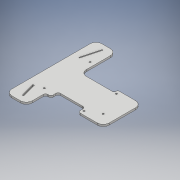
# Autodesk Inventor part: battery_mount
Saved by Autodesk Inventor 2017.2 (Build 212233000, 233)
## iProperties
Created: 2017-09-20
Part Number: battery_mount
Material: Generic
Document SubType Name: Modeling
Designer: Nic
Density: 1 g/cm^3
Appearance: Default
Author: Nic
Autodesk Inventor part; units mm, degrees
ref_plane "YZ Plane" through (0, 0, 0) normal (1, 0, 0) x (0, 1, 0)
ref_plane "XZ Plane" through (0, 0, 0) normal (0, 1, 0) x (-1, 0, 0)
ref_plane "XY Plane" through (0, 0, 0) normal (0, 0, 1) x (1, 0, 0)
sketch "Sketch1" plane through (0, 0, 0) normal (0, 0, 1) x (1, 0, 0)
  line L0 (-34, 30) -> (-34, -100)
  line L1 (96, -68) -> (96, -24)
  line L2 (0, -10) -> (0, 30)
  line L3 (-10, 40) -> (-24, 40)
  circle A0 centre (78, -60) radius 1.3
  circle A1 centre (-7.65, 3.7) radius 1.3
  arc A2 (-24, 40) -> (-34, 30) centre (-24, 30) ccw
  arc A3 (0, 30) -> (-10, 40) centre (-10, 30) ccw
  arc A4 (86, -78) -> (96, -68) centre (86, -68) ccw
  line L4 (0, -82) -> (0, -100)
  line L5 (-10, -110) -> (-24, -110)
  arc A5 (-10, -110) -> (0, -100) centre (-10, -100) ccw
  arc A6 (-34, -100) -> (-24, -110) centre (-24, -100) ccw
  line L6 (59, -14) -> (86, -14)
  arc A7 (96, -24) -> (86, -14) centre (86, -24) ccw
  line L7 (54, -74) -> (54, -70)
  line L8 (50, -66) -> (13, -66)
  line L9 (9, -70) -> (9, -72)
  line L10 (5, -78) -> (4, -78)
  line L11 (58, -78) -> (86, -78)
  arc A8 (13, -66) -> (9, -70) centre (13, -70) ccw
  arc A9 (54, -74) -> (58, -78) centre (58, -74) ccw
  arc A10 (54, -70) -> (50, -66) centre (50, -70) ccw
  line L12 (-16.3182, -100.6212) -> (-22.7887, -76.473)
  line L13 (-22.7887, -76.473) -> (-20.4705, -75.8519)
  line L14 (-20.4705, -75.8519) -> (-14, -100)
  line L15 (-14, -100) -> (-16.3182, -100.6212)
  line L16 (-10, -100) -> (-24, -100) construction
  line L17 (-34, -35) -> (96, -35) construction
  line L18 (-15.5455, 32) -> (-23.8277, 1.0904)
  line L19 (-15.5455, 32) -> (-14, 31.5859)
  line L20 (-14, 31.5859) -> (-22.2822, 0.6763)
  line L21 (-22.2822, 0.6763) -> (-23.8277, 1.0904)
  line L22 (53, -20) -> (10, -20)
  line L23 (56, -17) -> (56, -17)
  arc A11 (53, -20) -> (56, -17) centre (53, -17) ccw
  arc A12 (59, -14) -> (56, -17) centre (59, -17) ccw
  arc A13 (0, -10) -> (10, -20) centre (10, -10) ccw
  line L24 (-10, 30) -> (-24, 30) construction
  circle A14 centre (60, -20) radius 1.3
  circle A15 centre (58, -72) radius 1.3
  line L25 (9, -72) -> (9, -74)
  arc A16 (5, -78) -> (9, -74) centre (5, -74) ccw
  arc A17 (4, -78) -> (0, -82) centre (4, -82) ccw
  circle A18 centre (-8, -72) radius 1.3
  line L26 (58, -72) -> (-8, -72) construction
  point P0 (0, 0)
  point P1 (-34, 40)
  point P2 (0, 40)
  point P3 (-34, -110)
  point P4 (96, -14)
  point P5 (9, -78)
  point P6 (0, -20)
  point P7 (54, -66)
  point P8 (9, -66)
  dimension "d2" = 2.6
  dimension "d4" = 18
  dimension "d5" = 40
  dimension "d7" = 34
  dimension "d10" = 26.35
  dimension "d14" = 10
  dimension "d23" = 10
  dimension "d25" = 17.7
  dimension "d27" = 45
  dimension "d29" = 64
  dimension "d31" = 32
  dimension "d32" = 12
  dimension "d33" = 130
  dimension "d36" = 4
  dimension "d38" = 2.4
  dimension "d39" = 75
  dimension "d42" = 42
  dimension "d46" = 1.6
  dimension "d48" = 6
  dimension "d49" = 3
  dimension "d50" = 10
  dimension "d51" = 75
  dimension "d52" = 32
  dimension "d55" = 8
  dimension "d56" = 14
  dimension "d57" = 25
  dimension "d58" = 14
  dimension "d59" = 40
  dimension "d60" = 18
  dimension "d61" = 20
  dimension "d62" = 12
  dimension "d63" = 20
  dimension "d64" = 100
  dimension "d65" = 4
  dimension "d66" = 60
  dimension "d67" = 4
  dimension "d68" = 66
  constraints: 54 end point, 29 tangent, 28 point on circle, 19 centre point, 19 point on line, 16 perpendicular, 11 equal radius, 4 vertical, 3 horizontal, 1 collinear, 1 midpoint
  measures "d2" diameter of A0
  measures "d4" distance from line of L1 A0.centre
  measures "d5" distance from line of L3 point (0, 0)
  measures "d7" distance of point (0, 40) point (-34, 40)
  measures "d10" distance from line of L0 A1.centre
  measures "d14" radius of A2
  measures "d23" radius of A7
  measures "d25" distance from line of L6 A1.centre
  measures "d27" distance of point (54, -66) point (9, -66)
  measures "d29" distance between parallel lines of L6 L10
  measures "d31" distance from line of L5.start L10
  measures "d32" distance between parallel lines of L11 L8
  measures "d33" distance between parallel lines of L0 L1
  measures "d36" radius of A9
  measures "d38" distance between parallel lines of L14 L12
  measures "d39" angle of L12 L16
  measures "d42" distance between parallel lines of L1 L7
  measures "d46" distance between parallel lines of L20 L18
  measures "d48" distance between parallel lines of L6 L22
  measures "d49" radius of A11
  measures "d50" radius of A13
  measures "d51" angle of L24 L18
  measures "d52" distance of L19.end L20.end
  measures "d55" distance from line of L3 L18.start
  measures "d56" distance from line of L2 L19.end
  measures "d57" distance of L12.start L12.end
  measures "d58" distance from line of L4 L14.end
  measures "d59" vertical distance of A14.centre A0.centre
  measures "d60" horizontal distance of A0.centre A14.centre
  measures "d61" horizontal distance of A0.centre L26.start
  measures "d62" vertical distance of A0.centre L26.start
  measures "d63" distance from line of L22 point (0, 0)
  measures "d64" distance from line of point (0, 0) L16
  measures "d65" radius of A16
  measures "d66" vertical distance of point (0, 0) A0.centre
  measures "d67" horizontal distance of A14.centre L23.start
  measures "d68" distance of L26.start L26.end
extrude "Extrusion1" add sketch "Sketch1" along normal blind 3.175
body "Solid1"
